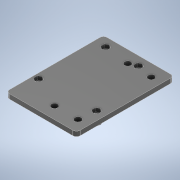
# Autodesk Inventor part: Electronics base
Saved by Autodesk Inventor 2022 (Build 260153000, 153)
## iProperties
Created: 2022-03-15
Part Number: Electronics base
Material: Genérico
Document SubType Name: Modeling
Designer: JK
Density: 1 g/cm^3
Appearance: Suave - Negro
Author: JK
Autodesk Inventor part; units mm, degrees
ref_plane "YZ Plane" through (0, 0, 0) normal (1, 0, 0) x (0, 1, 0)
ref_plane "XZ Plane" through (0, 0, 0) normal (0, 1, 0) x (-1, 0, 0)
ref_plane "XY Plane" through (0, 0, 0) normal (0, 0, 1) x (1, 0, 0)
sketch "Boceto1" plane through (0, 0, 0) normal (0, 1, 0) x (-1, 0, 0)
  line L0 (-30, 41.5) -> (30, 41.5)
  line L1 (30, 41.5) -> (30, -41.5)
  line L2 (30, -41.5) -> (-30, -41.5)
  line L3 (-30, -41.5) -> (-30, 41.5)
  line L4 (-30, 41.5) -> (30, -41.5) construction
  line L5 (30, 41.5) -> (-30, -41.5) construction
  circle A0 centre (-1, 31.2) radius 2.7
  circle A1 centre (-21, 31.2) radius 2.7
  circle A2 centre (-1, -31.2) radius 2.7
  circle A3 centre (-21, -31.2) radius 2.7
  point P0 (0, 0)
  dimension "d0" = 5.4
  dimension "d1" = 62.4
  dimension "d2" = 20
  dimension "d3" = 83
  dimension "d4" = 31.2
  dimension "d5" = 9
  dimension "d6" = 60
  constraints: 12 end point, 4 centre point, 3 equal radius, 2 horizontal alignment, 2 midpoint, 2 parallel, 2 vertical alignment, 1 horizontal, 1 perpendicular
  measures "d0" diameter of A0
  measures "d1" distance of A2.centre A0.centre
  measures "d2" distance of A0.centre A1.centre
  measures "d3" distance of L0.end L1.end
  measures "d4" vertical distance of A0.centre point (0, 0)
  measures "d5" distance from line of A1.centre L3
  measures "d6" distance of L0.start L0.end
extrude "Extrusión1" add sketch "Boceto1" along normal blind 4
fillet "Empalme1" radius 3 4 edges at (-30, 2, 41.5) (30, 2, 41.5) (30, 2, -41.5) (-30, 2, -41.5)
sketch "Boceto2" plane through (0, 0, 0) normal (0, -1, 0) x (1, 0, 0)
  circle A0 centre (-20.6319, -33.9933) radius 1.75 projected
  circle A1 centre (7.3081, -33.9933) radius 1.75 projected
  circle A2 centre (22.5481, 16.8067) radius 1.75 projected
  circle A3 centre (-25.7119, 18.0767) radius 1.75 projected
  point P0 (0, 0)
extrude "Extrusión2" cut sketch "Boceto2" against normal through all
sketch "Boceto4" plane through (0, 0, 0) normal (0, -1, 0) x (1, 0, 0)
  circle A0 centre (-20.6319, -33.9933) radius 1.75 projected
  circle A1 centre (-20.6319, -33.9933) radius 3
  circle A2 centre (-25.7119, 18.0767) radius 1.75 projected
  circle A3 centre (-25.7119, 18.0767) radius 3
  circle A4 centre (22.5481, 16.8067) radius 1.75 projected
  circle A5 centre (22.5481, 16.8067) radius 3
  circle A6 centre (21, -31.2) radius 2.7 projected
  circle A7 centre (7.3081, -33.9933) radius 1.75 projected
  circle A8 centre (7.3081, -33.9933) radius 3
  point P0 (0, 0)
  dimension "d12" = 6
  dimension "d16" = 6
  constraints: 4 centre point, 4 coincident, 2 equal radius
  measures "d12" diameter of A1
  measures "d16" diameter of A8
extrude "Extrusión3" add sketch "Boceto4" along normal blind 5 contours A1 | A3 | A5 | A8
fillet "Empalme2" radius 3 4 edges at (-23.6319, 0, -33.9933) (-28.7119, 0, 18.0767) (19.5481, 0, 16.8067) (4.3081, 0, -33.9933)
sketch "Boceto5" plane through (0, 4, 0) normal (0, 1, 0) x (1, 0, 0)
  circle A0 centre (-25.7119, -18.0767) radius 1.75 projected
  circle A1 centre (-25.7119, -18.0767) radius 2.85
  circle A2 centre (22.5481, -16.8067) radius 1.75 projected
  circle A3 centre (22.5481, -16.8067) radius 2.85
  circle A4 centre (-20.6319, 33.9933) radius 1.75 projected
  circle A5 centre (-20.6319, 33.9933) radius 2.85
  circle A6 centre (7.3081, 33.9933) radius 1.75 projected
  circle A7 centre (7.3081, 33.9933) radius 2.85
  line L0 (-25.7119, -14.7858) -> (-22.8619, -16.4313)
  line L1 (-22.8619, -16.4313) -> (-22.8619, -19.7221)
  line L2 (-22.8619, -19.7221) -> (-25.7119, -21.3676)
  line L3 (-25.7119, -21.3676) -> (-28.5619, -19.7221)
  line L4 (-28.5619, -19.7221) -> (-28.5619, -16.4313)
  line L5 (-28.5619, -16.4313) -> (-25.7119, -14.7858)
  line L6 (-20.6319, 37.2842) -> (-17.7819, 35.6387)
  line L7 (-17.7819, 35.6387) -> (-17.7819, 32.3479)
  line L8 (-17.7819, 32.3479) -> (-20.6319, 30.7024)
  line L9 (-20.6319, 30.7024) -> (-23.4819, 32.3479)
  line L10 (-23.4819, 32.3479) -> (-23.4819, 35.6387)
  line L11 (-23.4819, 35.6387) -> (-20.6319, 37.2842)
  line L12 (7.3081, 37.2842) -> (10.1581, 35.6387)
  line L13 (10.1581, 35.6387) -> (10.1581, 32.3479)
  line L14 (10.1581, 32.3479) -> (7.3081, 30.7024)
  line L15 (7.3081, 30.7024) -> (4.4581, 32.3479)
  line L16 (4.4581, 32.3479) -> (4.4581, 35.6387)
  line L17 (4.4581, 35.6387) -> (7.3081, 37.2842)
  line L18 (22.5481, -13.5158) -> (25.3981, -15.1613)
  line L19 (25.3981, -15.1613) -> (25.3981, -18.4521)
  line L20 (25.3981, -18.4521) -> (22.5481, -20.0976)
  line L21 (22.5481, -20.0976) -> (19.6981, -18.4521)
  line L22 (19.6981, -18.4521) -> (19.6981, -15.1613)
  line L23 (19.6981, -15.1613) -> (22.5481, -13.5158)
  point P0 (0, 0)
  dimension "d17" = 5.7
  constraints: 48 end point, 8 coincident, 4 centre point, 4 tangent, 4 vertical, 3 equal radius, 52 other
  measures "d17" diameter of A1
extrude "Extrusión4" cut sketch "Boceto5" against normal blind 3.1 contours A0 | A1 | L1 L2 A1 | A1 L0 L1 | A1 L5 L0 | L2 L3 A1 | A1 L4 L5 | L3 L4 A1 | A2 | A3 | L19 L20 A3 | A3 L18 L19 | A3 L23 L18 | L20 L21 A3 | A3 L22 L23 | L21 L22 A3 | A4 | A5 | L7 L8 A5 | A5 L6 L7 | A5 L11 L6 | L8 L9 A5 | A5 L10 L11 | L9 L10 A5 | A6 | A7 | L13 L14 A7 | A7 L12 L13 | A7 L17 L12 | L14 L15 A7 | A7 L16 L17 | L15 L16 A7
